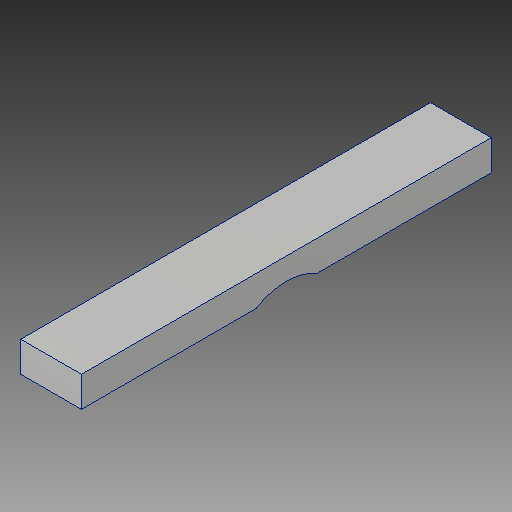
# Autodesk Inventor part: connectingthing
Saved by Autodesk Inventor 2017 (Build 210142000, 142)
## iProperties
Created: 2018-01-20
Part Number: connectingthing
Material: Aluminum 6061
Document SubType Name: Modeling
Designer: S331461152
Density: 2.7 g/cm^3
Appearance: Aluminum - Flat
Author: S331461152
Autodesk Inventor part; units mm, degrees
ref_plane "YZ Plane" through (0, 0, 0) normal (1, 0, 0) x (0, 1, 0)
ref_plane "XZ Plane" through (0, 0, 0) normal (0, 1, 0) x (-1, 0, 0)
ref_plane "XY Plane" through (0, 0, 0) normal (0, 0, 1) x (1, 0, 0)
sketch "Sketch1" plane through (0, 0, 0) normal (0, 0, 1) x (1, 0, 0)
  line L0 (0, 0) -> (0, -25.4)
  line L1 (0, -25.4) -> (50.8, -25.4)
  line L2 (50.8, -25.4) -> (50.8, 0)
  line L3 (50.8, 0) -> (0, 0)
  dimension "d0" = 25.4
  dimension "d1" = 50.8
  constraints: 8 end point, 3 perpendicular, 1 vertical
  measures "d0" distance of L0.start L0.end
  measures "d1" distance of L0.end L1.end
extrude "Extrusion1" add sketch "Sketch1" along normal blind 342.9
sketch "Sketch3" plane through (50.8, -25.4, 0) normal (1, 0, 0) x (0, 0, -1)
  line L0 (0, 0) -> (-342.9, 0) projected
  line L1 (-171.45, 0) -> (-196.8396, 0)
  line L2 (-196.8396, 0) -> (-146.0396, 0)
  arc A0 (-146.0396, 0) -> (-196.8396, 0) centre (-171.4396, -41.9008) ccw
  line L3 (-171.45, 0) -> (-171.45, 25.4)
  point P0 (0, 25.4)
  dimension "d10" = 50.8
  constraints: 6 end point, 2 point on circle, 2 point on line, 1 centre point, 1 midpoint, 1 vertical
  measures "d10" distance of L1.end L2.end
extrude "Extrusion2" cut sketch "Sketch3" against normal through all
body "Solid1"
